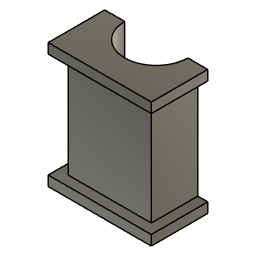
Excercise-3 by Chaitanya Sharma_ (Autodesk Fusion 360 design; units mm, degrees)
Autodesk Fusion 360 part; units mm, degrees
sketch "Sketch1" plane through (0, 0, 0) normal (0, 1, 0) x (1, 0, 0)
  line L0 (31, 37.5) -> (-31, 37.5)
  line L1 (-31, 37.5) -> (-31, -37.5)
  line L2 (-31, -37.5) -> (31, -37.5)
  line L3 (31, -37.5) -> (31, 37.5)
  constraint horizontal L0
  constraint perpendicular L0 L1
  constraint parallel L0 L2
  constraint parallel L1 L3
extrude "Extrude1" add sketch "Sketch1" along normal blind 34
sketch "Sketch2" plane through (0, 0, 37.5) normal (0, 0, 1) x (-1, 0, 0)
  line L0 (31, 0) -> (-31, 0)
  line L1 (-31, 0) -> (-31, -34)
  line L2 (-31, -34) -> (31, -34)
  line L3 (31, -34) -> (31, 0)
  arc A0 (19, -34) -> (-19, -34) centre (0, -34) ccw
  line L4 (19, -34) -> (-19, -34)
  dimension "d7" = 38
  constraint midpoint L2 A0.centre
  constraint coincident L2 A0.end
  constraint coincident L2 A0.start
  measures "d7" diameter of A0
extrude "Extrude2" cut sketch "Sketch2" against normal blind 75 contours L2 A0 L4
sketch "Sketch3" plane through (0, 34, 0) normal (0, 1, 0) x (-1, 0, 0)
  line L0 (19, 37.5) -> (19, -37.5)
  line L1 (19, -37.5) -> (31, -37.5)
  line L2 (31, -37.5) -> (31, 37.5)
  line L3 (31, 37.5) -> (19, 37.5)
  line L4 (31, -37.5) -> (31, -31.5)
  line L5 (31, -31.5) -> (25, -31.5)
  line L6 (31, 37.5) -> (31, 31.5)
  line L7 (31, 31.5) -> (25, 31.5)
  line L8 (25, 31.5) -> (25, -31.5)
  line L9 (0.133, -37.5) -> (0.133, 37.506)
  line L10 (-30.734, -31.5) -> (-24.734, -31.5)
  line L11 (-24.734, 31.5) -> (-24.734, -31.5)
  line L12 (-30.734, 31.5) -> (-24.734, 31.5)
  dimension "d10" = 6
  dimension "d11" = 6
  dimension "d12" = 6
  dimension "d13" = 6
  constraint coincident L1.end L2.start
  constraint perpendicular L1 L4
  constraint perpendicular L2 L5
  constraint coincident L2.end L3.start
  constraint perpendicular L3 L6
  constraint perpendicular L2 L7
  constraint perpendicular L1 L9
  constraint symmetric L4.end L9 L10.start
  constraint symmetric L5.end L9 L10.end
  constraint symmetric L6.end L9 L12.start
  constraint symmetric L7.end L9 L11.start
  measures "d10" distance of L1.end L4.end
  measures "d11" distance of L4.end L5.end
  measures "d12" distance of L2.end L6.end
  measures "d13" distance of L6.end L7.end
extrude "Extrude3" cut sketch "Sketch3" against normal blind 34 contours L2 L5 L7 L8
sketch "Sketch4" plane through (0, 34, 0) normal (0, 1, 0) x (-1, 0, 0)
  line L0 (-19, -37.5) -> (-19, 37.5)
  line L1 (-19, 37.5) -> (-31, 37.5)
  line L2 (-31, 37.5) -> (-31, -37.5)
  line L3 (-31, -37.5) -> (-19, -37.5)
  line L4 (-31, -37.5) -> (-31, -31.5)
  line L5 (-31, -31.5) -> (-25, -31.5)
  line L6 (-31, 37.5) -> (-31, 31.5)
  line L7 (-31, 31.5) -> (-25, 31.5)
  line L8 (-25, 31.5) -> (-25, -31.5)
  dimension "d16" = 6
  dimension "d17" = 6
  dimension "d18" = 6
  dimension "d19" = 6
  constraint coincident L2.end L3.start
  constraint perpendicular L3 L4
  constraint perpendicular L4 L5
  constraint coincident L1.end L2.start
  constraint perpendicular L1 L6
  constraint perpendicular L2 L7
  measures "d16" distance of L2.end L4.end
  measures "d17" distance of L4.end L5.end
  measures "d18" distance of L1.end L6.end
  measures "d19" distance of L6.end L7.end
extrude "Extrude4" cut sketch "Sketch4" against normal blind 34 contours L2 L5 L7 L8
sketch "Sketch5" plane through (25, 0, 0) normal (1, 0, 0) x (0, 1, 0)
  line L0 (34, -31.5) -> (34, 31.5)
  line L1 (34, 31.5) -> (0, 31.5)
  line L2 (0, 31.5) -> (0, -31.5)
  line L3 (0, -31.5) -> (34, -31.5)
  line L4 (0, -31.5) -> (6, -31.5)
  line L5 (6, -31.5) -> (6, 31.5)
  dimension "d22" = 6
  constraint coincident L2.end L3.start
  constraint perpendicular L2 L4
  constraint coincident L1 L5.end
  constraint perpendicular L1 L5
  measures "d22" distance of L2.end L4.end
extrude "Extrude5" cut sketch "Sketch5" against normal blind 50 contours L1 L2 L3 L4 L5
